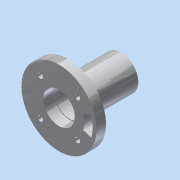
# Autodesk Inventor part: StatorCore
Saved by Autodesk Inventor 2015 (Build 190159000, 159)
## iProperties
Created: 2015-12-24
Part Number: StatorCore
Material: Aluminum 6061
Document SubType Name: Modeling
Designer: Raphael
Density: 2.7 g/cm^3
Appearance: Aluminum - Flat
Author: Raphael
Autodesk Inventor part; units mm, degrees
ref_plane "YZ Plane" through (0, 0, 0) normal (1, 0, 0) x (0, 1, 0)
ref_plane "XZ Plane" through (0, 0, 0) normal (0, 1, 0) x (-1, 0, 0)
ref_plane "XY Plane" through (0, 0, 0) normal (0, 0, 1) x (1, 0, 0)
sketch "Sketch1" plane through (0, 0, 0) normal (1, 0, 0) x (0, 1, 0)
  line L0 (0, 0) -> (25, 0)
  line L1 (25, 0) -> (25, -6.35)
  line L2 (25, -6.35) -> (11.5, -6.35)
  line L3 (11.5, -6.35) -> (11.5, -41.35)
  line L4 (11.5, -41.35) -> (10.5, -41.35)
  line L5 (10.5, -41.35) -> (10.5, -37.35)
  line L6 (10.5, -37.35) -> (10, -37.35)
  line L7 (10, -37.35) -> (10, -7.175)
  line L8 (10, -7.175) -> (10.5, -7.175)
  line L9 (10.5, -7.175) -> (10.5, 0)
  line L10 (0, -49.62) -> (0, 8.27) projected
  dimension "d0" = 25
  dimension "d1" = 6.35
  dimension "d4" = 35
  dimension "d5" = 4
  dimension "d6" = 7.175
  dimension "d7" = 10.5
  dimension "d9" = 0.5
  dimension "d11" = 11.5
  constraints: 20 end point, 6 perpendicular, 3 point on line, 2 horizontal, 1 vertical
  measures "d0" distance of L0.start L0.end
  measures "d1" distance of L0.end L1.end
  measures "d4" distance of L2.end L3.end
  measures "d5" distance of L4.end L5.end
  measures "d6" distance of L8.end L9.end
  measures "d7" distance from line of L0.start L5
  measures "d9" distance between parallel lines of L5 L7
  measures "d11" distance between parallel lines of L10 L3
derived "Stator.ipt"
revolve "Revolution1" add sketch "Sketch1" angle 360 about axis through (0, 0, -10) along (0, 0, 1)
sketch "Sketch2" plane through (0, 0, 0) normal (0, 0, 1) x (1, 0, 0)
  arc A0 (21.5281, -6.3543) -> (21.5281, 6.3543) centre (0, 0) ccw
  arc A1 (16.2191, -4.6606) -> (16.2191, 4.6606) centre (0, 0) ccw
  line L0 (21.5281, 6.3543) -> (16.2191, 4.6606)
  line L1 (21.5281, -6.3543) -> (16.2191, -4.6606)
  line L2 (-35, 0) -> (35, 0) projected
  circle A2 centre (-12.3744, 12.3744) radius 1.75
  line L3 (0, 0) -> (-12.3744, 12.3744) construction
  circle A3 centre (0, 0) radius 10 projected
  circle A4 centre (0, 0) radius 25 projected
  line L4 (-12.3744, 12.3744) -> (-17.6777, 17.6777) construction
  circle A5 centre (0, 0) radius 25 projected
  line L5 (-12.3744, 12.3744) -> (-7.0711, 7.0711) construction
  circle A6 centre (-12.3744, -12.3744) radius 1.75
  circle A7 centre (12.3744, -12.3744) radius 1.75
  circle A8 centre (12.3744, 12.3744) radius 1.75
  dimension "d12" = 3.5
  dimension "d15" = 45
  dimension "d19" = 360
  constraints: 10 end point, 6 centre point, 5 point on circle, 3 collinear, 2 coincident, 16 other
  measures "d12" diameter of A2
  measures "d15" angle of L2 L3
extrude "Extrusion1" cut sketch "Sketch2" against normal through all contours L1 A1 L2 A0 | L2 A1 L0 A0 | A2 | A6 | A7 | A8
equation "\"d11\" = 0.5 * stator_id"
equation "\"stator_id\" = 23"
body "Solid1"
